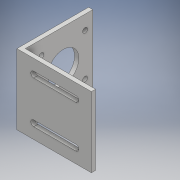
# Autodesk Inventor part: 모터 브라켓
Saved by Autodesk Inventor 2018 (Build 220112000, 112)
## iProperties
Created: 2019-01-29
Part Number: 모터 브라켓
Material: Generic
Document SubType Name: Modeling
Designer: User
Density: 1 g/cm^3
Appearance: Default
Author: User
Autodesk Inventor part; units mm, degrees
ref_plane "YZ Plane" through (0, 0, 0) normal (1, 0, 0) x (0, 1, 0)
ref_plane "XZ Plane" through (0, 0, 0) normal (0, 1, 0) x (-1, 0, 0)
ref_plane "XY Plane" through (0, 0, 0) normal (0, 0, 1) x (1, 0, 0)
sketch "스케치1" plane through (0, 0, 0) normal (1, 0, 0) x (0, 1, 0)
  line L0 (0, 0) -> (51, 0)
  line L1 (51, 0) -> (51, -50)
  line L2 (51, -50) -> (0, -50)
  line L3 (0, -50) -> (0, 0)
  line L4 (0, -25) -> (30, -25)
  line L5 (0, -10) -> (14.5, -10)
  line L6 (0, -40) -> (14.5, -40)
  line L7 (14.5, -10) -> (45.5, -10)
  line L8 (14.5, -40) -> (45.5, -40)
  circle A0 centre (45.5, -10) radius 1.75
  circle A1 centre (14.5, -10) radius 1.75
  circle A2 centre (45.5, -40) radius 1.75
  circle A3 centre (14.5, -40) radius 1.75
  circle A4 centre (30, -25) radius 11.05
  line L9 (3, -50) -> (3, 0)
  dimension "d0" = 51
  dimension "d1" = 50
  dimension "d2" = 30
  dimension "d3" = 14.5
  dimension "d4" = 14.5
  dimension "d5" = 31
  dimension "d6" = 31
  dimension "d7" = 3.5
  dimension "d8" = 3.5
  dimension "d9" = 3.5
  dimension "d10" = 3.5
  dimension "d11" = 22.1
  constraints: 20 end point, 6 horizontal, 5 centre point, 5 coincident, 5 point on line, 2 parallel, 2 perpendicular, 1 midpoint
  measures "d0" distance of L1.end L2.end
  measures "d1" distance of L0.end L1.end
  measures "d2" distance of L4.start L4.end
  measures "d3" distance of L5.start L5.end
  measures "d4" distance of L6.start L6.end
  measures "d5" distance of L5.end L7.end
  measures "d6" distance of L6.end L8.end
  measures "d7" diameter of A0
  measures "d8" diameter of A1
  measures "d9" diameter of A2
  measures "d10" diameter of A3
  measures "d11" diameter of A4
extrude "돌출1" add sketch "스케치1" along normal blind 3 contours L0 L1 L2 L9
extrude "돌출2" add sketch "스케치1" along normal blind 53 contours L0 L9 L5 L3 | L5 L9 L4 L3 | L4 L9 L6 L3 | L6 L9 L2 L3
sketch "스케치2" plane through (0, 0, -50) normal (0, -1, 0) x (1, 0, 0)
  line L0 (53, 0) -> (53, 10)
  line L1 (53, 0) -> (53, 50) projected
  line L2 (53, 10) -> (42, 10)
  line L3 (53, 50) -> (53, 40)
  line L4 (53, 40) -> (42, 40)
  arc A0 (12, 12.1) -> (12, 7.9) centre (12, 10) ccw
  arc A1 (42, 7.9) -> (42, 12.1) centre (42, 10) ccw
  arc A2 (12, 42.1) -> (12, 37.9) centre (12, 40) ccw
  arc A3 (42, 37.9) -> (42, 42.1) centre (42, 40) ccw
  line L5 (12, 12.1) -> (42, 12.1)
  line L6 (12, 37.9) -> (42, 37.9)
  line L7 (42, 42.1) -> (12, 42.1)
  line L8 (12, 7.9) -> (42, 7.9)
  point P0 (0, 50)
  dimension "d16" = 10
  dimension "d17" = 11
  dimension "d18" = 10
  dimension "d19" = 11
  dimension "d22" = 4.2
  dimension "d23" = 4.2
  dimension "d24" = 4.2
  dimension "d25" = 4.2
  constraints: 16 end point, 8 point on circle, 4 centre point, 3 parallel, 2 coincident, 2 perpendicular, 2 point on line, 1 horizontal, 1 tangent
  measures "d16" distance of L0.start L0.end
  measures "d17" distance of L0.end L2.end
  measures "d18" distance of L1.end L3.end
  measures "d19" distance of L3.end L4.end
  measures "d22" diameter of A0
  measures "d23" diameter of A1
  measures "d24" diameter of A2
  measures "d25" diameter of A3
extrude "돌출3" cut sketch "스케치2" against normal blind 3
